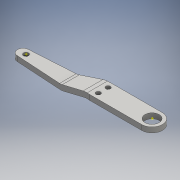
# Autodesk Inventor part: Profile_Straight_05
Saved by Autodesk Inventor 2016 (Build 200138000, 138)
## iProperties
Created: 2016-02-08
Part Number: Profile_Straight_05
Material: Generic
Document SubType Name: Modeling
Designer: nils
Density: 1 g/cm^3
Appearance: Default
Mass: 684.21 g
Surface Area: 1010.33 cm^2
Volume: 684.21 cm^3
Author: nils
Autodesk Inventor part; units mm, degrees
ref_plane "YZ Plane" through (0, 0, 0) normal (1, 0, 0) x (0, 1, 0)
ref_plane "XZ Plane" through (0, 0, 0) normal (0, 1, 0) x (-1, 0, 0)
ref_plane "XY Plane" through (0, 0, 0) normal (0, 0, 1) x (1, 0, 0)
sketch "Sketch4" plane through (0, 0, 0) normal (1, 0, 0) x (0, 1, 0)
  line L0 (-40, 10) -> (40, 10)
  line L1 (40, 10) -> (40, -10)
  line L2 (40, -10) -> (-40, -10)
  line L3 (-40, -10) -> (-40, 10)
  line L4 (-40, 10) -> (40, -10) construction
  line L5 (40, 10) -> (-40, -10) construction
  point P0 (0, 0)
  dimension "d15" = 20
  dimension "d16" = 80
  constraints: 12 end point, 2 midpoint, 2 parallel, 1 horizontal, 1 perpendicular
  measures "d15" distance between parallel lines of L2 L0
  measures "d16" distance of L1.end L2.end
sketch "Sketch5" plane through (0, 0, 0) normal (0, 1, 0) x (-1, 0, 0)
  line L0 (0, 0) -> (220, 0)
  line L1 (220, 0) -> (320, -28.8125)
  line L2 (320, -28.8125) -> (490, -28.8125)
  dimension "d17" = 490
  dimension "d18" = 220
  dimension "d19" = 320
  constraints: 6 end point, 1 horizontal, 1 parallel
  measures "d17" horizontal distance of L0.start L2.end
  measures "d18" distance of L0.start L0.end
  measures "d19" horizontal distance of L0.start L1.end
sweep "Sweep1" add profiles "Sketch4" path "Sketch5"
sketch "Sketch9" plane through (0, -40, 10) normal (1, 0, 0) x (0, 0, -1)
  line L0 (0, 0) -> (0, 80) projected
  line L1 (20, 0) -> (0, 0) projected
  line L2 (0, 80) -> (20, 80)
  line L3 (20, 80) -> (20, 0)
  line L4 (20, 0) -> (0, 0)
  line L5 (0, 0) -> (0, 80)
  point P0 (10, 40)
  constraints: 8 end point, 2 parallel, 1 horizontal, 1 perpendicular
extrude "Extrusion2" add sketch "Sketch9" along normal blind 40
sketch "Sketch10" plane through (-490, -40, -18.8125) normal (-1, 0, 0) x (0, 0, 1)
  line L0 (8.8125, 80) -> (-20, 80) projected
  line L1 (0, 0) -> (0, 80) projected
  line L2 (-20, 80) -> (0, 80)
  line L3 (0, 80) -> (0, 0)
  line L4 (0, 0) -> (-20, 0)
  line L5 (-20, 0) -> (-20, 80)
  point P0 (18.8125, 40)
  constraints: 8 end point, 2 parallel, 1 horizontal, 1 perpendicular
extrude "Extrusion3" add sketch "Sketch10" along normal blind 32.5
hole "Hole1" at (0, 0, 10) direction (0, 0, -1) diameter 55 end through all
hole "Hole2" at (-490, 0, -18.8125) direction (0, 0, -1) diameter 20 end through all
sketch "Sketch12" plane through (-318.5881, -40, -38.8125) normal (0, 0, -1) x (-1, 0, 0)
  line L0 (151.4119, 25) -> (191.4119, 25)
  line L1 (191.4119, 25) -> (191.4119, 55)
  line L2 (191.4119, 55) -> (151.4119, 55)
  line L3 (151.4119, 55) -> (151.4119, 25)
  line L4 (151.4119, 25) -> (191.4119, 55) construction
  line L5 (191.4119, 25) -> (151.4119, 55) construction
  line L6 (0, 0) -> (203.9119, 0) projected
  point P0 (-318.5881, 40)
  point P1 (171.4119, 40)
  dimension "d44" = 40
  dimension "d45" = 30
  dimension "d46" = 40
  dimension "d47" = 490
  constraints: 12 end point, 2 midpoint, 2 parallel, 1 horizontal, 1 perpendicular
  measures "d44" distance of L1.end L2.end
  measures "d45" distance of L0.end L1.end
  measures "d46" distance from line of L6 point (171.412, 40)
  measures "d47" distance of point (171.412, 40) point (-318.588, 40)
extrude "Extrusion4" cut sketch "Sketch12" against normal blind 10
fillet "Fillet1" radius 40 2 edges at (-218.5881, 0, -10) (-321.4119, 0, -18.8125)
fillet "Fillet2" radius 60 2 edges at (-221.4119, 0, 10) (-318.5881, 0, -38.8125)
fillet "Fillet3" radius 40 2 edges at (40, 40, 0) (40, -40, 0)
fillet "Fillet4" radius 8 4 edges at (-470, 15, -33.8125) (-510, 15, -33.8125) (-470, -15, -33.8125) (-510, -15, -33.8125)
sketch "Sketch15" plane through (-522.5, -40, -38.8125) normal (0, 0, -1) x (-1, 0, 0)
  line L0 (0, 0) -> (0, 80) projected
  line L1 (0, 60) -> (-320, 80)
  line L2 (-522.5, 80) -> (-309.5595, 80) projected
  line L3 (-195.4405, 80) -> (0, 80) projected
  line L4 (0, 80) -> (-320, 80)
  line L5 (0, 80) -> (0, 60)
  line L6 (0, 20) -> (-320, 0)
  line L7 (-522.5, 0) -> (-309.5595, 0) projected
  line L8 (-195.4405, 0) -> (0, 0) projected
  line L9 (0, 0) -> (0, 20)
  line L10 (-320, 80) -> (-320, 0) construction
  line L11 (-320, 0) -> (0, 0)
  point P0 (-522.5, 40)
  dimension "d73" = 20
  dimension "d74" = 40
  dimension "d75" = 320
  constraints: 14 end point, 4 point on line, 3 collinear, 1 horizontal, 1 perpendicular
  measures "d73" distance from line of L3 L1.start
  measures "d74" distance of L6.start L1.start
  measures "d75" distance between parallel lines of L0 L10
extrude "Extrusion6" cut sketch "Sketch15" against normal through all
fillet "Fillet7" radius 20 2 edges at (-522.5, -20, -28.8125) (-522.5, 20, -28.8125)
sketch "Sketch20" plane through (40, -5, -10) normal (0, 0, -1) x (-1, 0, 0)
  line L0 (562.5, 3.789) -> (562.5, 6.211) projected
  circle A0 centre (40, 5) radius 27.5 projected
  line L1 (242.5, -35) -> (40, -35) projected
  line L2 (230, -35) -> (230, 45)
  line L3 (40, 45) -> (242.5, 45) projected
  point P0 (230, -14)
  point P1 (230, 24)
  dimension "d140" = 190
  dimension "d141" = 21
  dimension "d142" = 21
  constraints: 4 point on line, 2 end point, 1 vertical
  measures "d140" distance from line of A0.centre L2
  measures "d141" distance from line of L1 point (230, -14)
  measures "d142" distance from line of L3 point (230, 24)
hole "Hole7" at (-190, -19, -10) at (-190, 19, -10) direction (0, 0, 1) diameter 17.5 end through all countersink diameter 34 countersink angle 90
body "Solid2"
